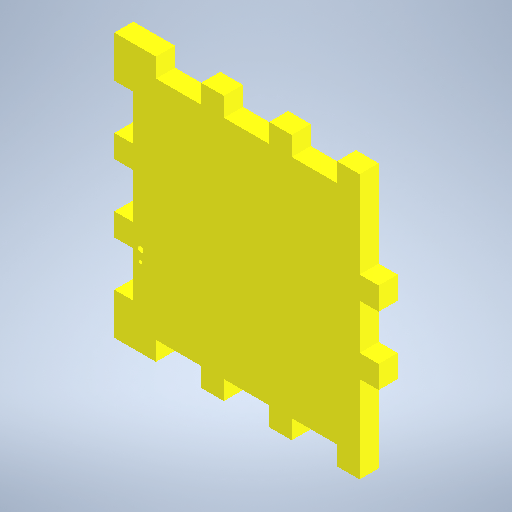
# Autodesk Inventor part: 5
Saved by Autodesk Inventor 2025.3 (Build 293356000, 356)
## iProperties
Created: 2025-12-22
Part Number: 5
Material: Generic
Document SubType Name: Sheet Metal
Designer: Balint
Density: 1 g/cm^3
Sheet Metal Rule: Default_mm
Appearance: Default
Flat Pattern Width: 25 cm
Flat Pattern Length: 25 cm
Flat Pattern Area: 625 cm^2
Sheet Metal Width: 250.000 mm
Sheet Metal Length: 250.000 mm
Sheet Metal Area: 62500.000 mm^2
Author: Balint
Autodesk Inventor part; units mm, degrees
ref_plane "YZ Plane" through (0, 0, 0) normal (1, 0, 0) x (0, 1, 0)
ref_plane "XZ Plane" through (0, 0, 0) normal (0, 1, 0) x (-1, 0, 0)
ref_plane "XY Plane" through (0, 0, 0) normal (0, 0, 1) x (1, 0, 0)
sketch "Sketch1" plane through (0, 0, 0) normal (0, 0, 1) x (1, 0, 0)
  line L0 (-210.6, 18) -> (39.4, 18)
  line L1 (39.4, 18) -> (39.4, -232)
  line L2 (39.4, -232) -> (-210.6, -232)
  line L3 (-210.6, -232) -> (-210.6, 18)
  line L4 (21.4, -214) -> (21.4, 0)
  line L5 (21.4, -214) -> (-192.6, -214)
  line L6 (-192.6, -214) -> (21.4, -214)
  line L7 (39.4, 0) -> (39.4, -21.4)
  line L8 (39.4, -21.4) -> (21.4, -21.4)
  line L9 (21.4, -21.4) -> (21.4, 0)
  line L10 (39.4, -64.2) -> (21.4, -64.2)
  line L11 (21.4, -64.2) -> (21.4, -85.6)
  line L12 (21.4, -85.6) -> (39.4, -85.6)
  line L13 (21.4, -128.4) -> (39.4, -128.4)
  line L14 (39.4, -149.8) -> (21.4, -149.8)
  line L15 (39.4, -192.6) -> (21.4, -192.6)
  line L16 (-210.6, 18) -> (-210.6, 0)
  line L17 (21.4, 0) -> (21.4, 18)
  line L18 (-210.6, -192.6) -> (-192.6, -192.6)
  line L19 (-210.6, -149.8) -> (-192.6, -149.8)
  line L20 (-192.6, -128.4) -> (-210.6, -128.4)
  line L21 (-192.6, -85.6) -> (-210.6, -85.6)
  line L22 (-210.6, -64.2) -> (-192.6, -64.2)
  line L23 (-210.6, -21.4) -> (-192.6, -21.4)
  line L24 (-64.2, -214) -> (-64.2, -232)
  line L25 (-107, -214) -> (-107, -232)
  line L26 (-128.4, -232) -> (-128.4, -214)
  line L27 (-171.2, -232) -> (-171.2, -214)
  line L28 (-42.8, -232) -> (-42.8, -214)
  line L29 (0, -232) -> (0, -214)
  line L30 (-64.2, 18) -> (-64.2, 0)
  line L31 (-42.8, 0) -> (-42.8, 18)
  line L32 (0, 0) -> (0, 18)
  line L33 (-128.4, 0) -> (-128.4, 18)
  line L34 (-171.2, 0) -> (-171.2, 18)
  line L35 (-107, 18) -> (-107, 0)
  line L36 (21.4, 0) -> (-192.6, 0)
  line L37 (-192.6, 0) -> (-192.6, -214)
  line L38 (21.4, -214) -> (21.4, -232)
  point P0 (0, 0)
  point P1 (227.0923, 209.5253)
  point P2 (245.0923, 209.5253)
  point P3 (227.0923, 252.3253)
  point P4 (205.6923, 273.7253)
  point P5 (205.6923, 291.7253)
  point P6 (162.8923, 291.7253)
  point P7 (162.8923, 273.7253)
  point P8 (141.4923, 273.7253)
  point P9 (141.4923, 291.7253)
  point P10 (98.6923, 291.7253)
  point P11 (98.6923, 273.7253)
  point P12 (77.2923, 273.7253)
  point P13 (77.2923, 291.7253)
  point P14 (34.4923, 291.7253)
  point P15 (34.4923, 273.7253)
  point P16 (13.0923, 252.3253)
  point P17 (-4.9077, 252.3253)
  point P18 (-4.9077, 209.5253)
  point P19 (13.0923, 209.5253)
  point P20 (13.0923, 188.1253)
  point P21 (-4.9077, 188.1253)
  point P22 (-4.9077, 145.3253)
  point P23 (13.0923, 145.3253)
  point P24 (13.0923, 123.9253)
  point P25 (-4.9077, 123.9253)
  point P26 (-4.9077, 81.1253)
  point P27 (13.0923, 81.1253)
  point P28 (13.0923, 59.7253)
  point P29 (34.4923, 59.7253)
  point P30 (34.4923, 41.7253)
  point P31 (77.2923, 41.7253)
  point P32 (77.2923, 59.7253)
  point P33 (98.6923, 59.7253)
  point P34 (98.6923, 41.7253)
  point P35 (141.4923, 41.7253)
  point P36 (141.4923, 59.7253)
  point P37 (162.8923, 59.7253)
  point P38 (162.8923, 41.7253)
  point P39 (205.6923, 41.7253)
  point P40 (205.6923, 59.7253)
  point P41 (227.0923, 59.7253)
  point P42 (227.0923, 81.1253)
  point P43 (245.0923, 81.1253)
  point P44 (245.0923, 123.9253)
  point P45 (227.0923, 123.9253)
  point P46 (227.0923, 145.3253)
  point P47 (245.0923, 145.3253)
  point P48 (245.0923, 188.1253)
  point P49 (227.0923, 188.1253)
  point P50 (-210.6, -232)
  dimension "d0" = 250
  dimension "d1" = 250
  dimension "d2" = 21.4
  measures "d0" distance of L1.end L2.end
  measures "d1" distance of L0.end L1.end
  measures "d2" distance of L7.start L7.end
extrude "Plate1" add sketch "Sketch1" against normal blind 18 contours L0 L34 L36 L37 L23 L3 | L0 L35 L36 L33 | L36 L4 L5 L37 | L22 L37 L21 L3 | L0 L31 L36 L30 | L20 L37 L19 L3 | L0 L17 L36 L32 | L18 L37 L5 L27 L2 L3 | L10 L1 L12 L4 | L26 L5 L25 L2 | L13 L1 L14 L4 | L24 L5 L28 L2 | L29 L5 L38 L2
sketch "Sketch2" plane through (0, 0, -18) normal (0, 0, -1) x (-1, 0, 0)
  circle A0 centre (185.6, -157.4) radius 1.75
  line L0 (192.6, -137.4) -> (-21.4, -137.4) projected
  line L1 (192.6, -192.6) -> (192.6, -149.8) projected
  line L2 (210.6, -232) -> (171.2, -232) projected
  circle A1 centre (185.6, -146.9845) radius 2.75
  point P0 (0, 0)
  dimension "d4" = 3.5
  dimension "d5" = 20
  dimension "d6" = 7
  dimension "d7" = 5.5
  dimension "d8" = 7
  constraints: 2 centre point
  measures "d4" diameter of A0
  measures "d5" distance from line of L0 A0.centre
  measures "d6" distance from line of L1 A0.centre
  measures "d7" diameter of A1
  measures "d8" distance from line of L1 A1.centre
extrude "Cut1" cut sketch "Sketch2" against normal blind 18
equation "\"d9\" = Thickness"
equation "\"d3\" = Thickness"
equation "\"BendRadius\" = Thickness"
equation "\"BendReliefWidth\" = Thickness"
equation "\"BendReliefDepth\" = 0.5 * Thickness"
equation "\"CornerReliefSize\" = 4 * Thickness"
equation "\"MinimumRemnant\" = 2 * Thickness"
equation "\"TransitionRadius\" = BendRadius"
equation "\"JacobiRadiusSize\" = BendRadius"
equation "\"GapSize\" = Thickness"
equation "\"Thickness\" = 18"
body "Solid1"
